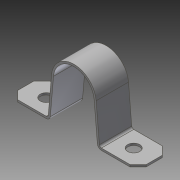
# Autodesk Inventor part: Pneumatics Steel Bracket
Saved by Autodesk Inventor 2014 SP1 (Build 180222100, 222)
## iProperties
Created: 2013-12-16
Part Number: Pneumatics Steel Bracket
Material: Steel
Document SubType Name: Modeling
Designer: Moses
Density: 7.85 g/cm^3
Appearance: Steel
Mass: 6.47227 g
Surface Area: 22.5229 cm^2
Volume: 0.824493 cm^3
Author: Moses
Autodesk Inventor part; units mm, degrees
ref_plane "YZ Plane" through (0, 0, 0) normal (1, 0, 0) x (0, 1, 0)
ref_plane "XZ Plane" through (0, 0, 0) normal (0, 1, 0) x (-1, 0, 0)
ref_plane "XY Plane" through (0, 0, 0) normal (0, 0, 1) x (1, 0, 0)
sketch "Sketch1" plane through (0, 0, 0) normal (0, 0, 1) x (1, 0, 0)
  line L0 (0, 0) -> (14.4203, 0)
  line L1 (16.0018, 1.4491) -> (17.2586, 15.8146)
  arc A0 (33.2345, 15.8146) -> (17.2586, 15.8146) centre (25.2465, 15.1157) ccw
  line L2 (33.2345, 15.8146) -> (34.4913, 1.4491)
  line L3 (36.0728, 0) -> (50.4931, 0)
  arc A1 (14.4203, 0) -> (16.0018, 1.4491) centre (14.4203, 1.5875) ccw
  arc A2 (34.4913, 1.4491) -> (36.0728, 0) centre (36.0728, 1.5875) ccw
  line L4 (0, 0.7937) -> (14.4203, 0.7937)
  arc A3 (14.4203, 0.7937) -> (15.2111, 1.5183) centre (14.4203, 1.5875) ccw
  line L5 (15.2111, 1.5183) -> (16.4679, 15.8838)
  arc A4 (34.0252, 15.8838) -> (16.4679, 15.8838) centre (25.2465, 15.1157) ccw
  line L6 (34.0252, 15.8838) -> (35.282, 1.5183)
  arc A5 (35.282, 1.5183) -> (36.0728, 0.7938) centre (36.0728, 1.5875) ccw
  line L7 (36.0728, 0.7938) -> (50.4931, 0.7938)
  line L8 (0, 0.7937) -> (0, 0)
  line L9 (50.4931, 0.7938) -> (50.4931, 0)
  line L10 (17.944, 18.4277) -> (32.549, 18.4277) construction
  point P0 (15.875, 0)
  dimension "d0" = 15.875
  dimension "d1" = 15.875
  dimension "d2" = 1.5875
  dimension "d3" = 95
  dimension "d4" = 95
  dimension "d6" = 0.7937
  dimension "d18" = 14.605
  dimension "d19" = 18.4277
  constraints: 22 end point, 14 point on circle, 6 centre point, 6 tangent, 2 collinear, 2 equal length, 2 horizontal, 2 point on line, 2 vertical, 1 equal radius, 6 other
  measures "d0" distance of L0.start point (15.875, 0)
  measures "d1" distance of point (15.875, 0) L1.end
  measures "d2" radius of A1
  measures "d3" angle of L1 L0
  measures "d4" angle of L3 L2
  measures "d6" distance of L7.end L3.end
  measures "d18" distance of L10.start L10.end
  measures "d19" distance between parallel lines of L3 L10
extrude "Extrusion1" add sketch "Sketch1" along normal blind 12.7
chamfer "Chamfer1" distance 3.175 angle 45 4 edges at (0, 0.3969, 12.7) (50.4931, 0.3969, 12.7) (50.4931, 0.3969, 0) (0, 0.3969, 0)
sketch "Sketch2" plane through (36.0728, 0, 0) normal (0, -1, 0) x (1, 0, 0)
  line L0 (0, 12.7) -> (11.2453, 12.7) projected
  line L1 (0, 0) -> (0, 12.7) projected
  line L2 (0, 0) -> (11.2453, 0) projected
  line L3 (-32.8978, 0) -> (-36.0728, 3.175) projected
  line L4 (-32.8978, 0) -> (-21.6524, 0) projected
  line L5 (-21.6524, 0) -> (-21.6524, 12.7) projected
  line L6 (-32.8978, 12.7) -> (-21.6524, 12.7) projected
  line L7 (-36.0728, 9.525) -> (-32.8978, 12.7) projected
  line L8 (-36.0728, 3.175) -> (-36.0728, 9.525) projected
  line L9 (6.35, 12.7) -> (6.35, 0) construction
  line L10 (-28.0024, 12.7) -> (-28.0024, 0) construction
  circle A0 centre (-28.0024, 6.35) radius 2.3813
  circle A1 centre (6.35, 6.35) radius 2.3813
  point P0 (-36.0728, 0)
  dimension "d12" = 4.7625
  dimension "d13" = 4.7625
  dimension "d14" = 6.35
  dimension "d15" = 6.35
  constraints: 4 end point, 4 point on line, 2 centre point, 2 midpoint, 2 vertical
  measures "d12" diameter of A0
  measures "d13" diameter of A1
  measures "d14" distance between parallel lines of L5 L10
  measures "d15" distance between parallel lines of L9 L1
extrude "Extrusion2" cut sketch "Sketch2" against normal through all contours A0 | A1
equation "\"d4\" = d3"
equation "\"d12\" = d13"
equation "\"d15\" = d14"
body "Solid1"
